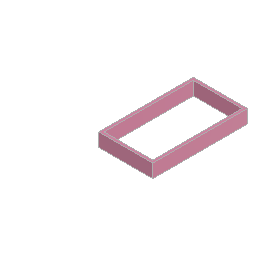
Digital-Storage-Holdster (Autodesk Fusion 360 design; units mm, degrees)
Autodesk Fusion 360 part; units mm, degrees
sketch "Sketch1" plane through (0, 0, 3.175) normal (0, 0, 1) x (-1, 0, 0)
  line L0 (0, 0) -> (0, 297.942)
  line L1 (0, 297.942) -> (-407.924, 297.942)
  line L2 (-407.924, 297.942) -> (-407.924, 0)
  line L3 (-407.924, 0) -> (0, 0)
  line L4 (0, 297.942) -> (-60, 297.942)
  line L5 (-60, 297.942) -> (-60, 192.942)
  line L6 (-60, 192.942) -> (0, 192.942)
  line L7 (0, 192.942) -> (0, 297.942)
  line L8 (-2.95, 294.992) -> (-57.05, 294.992)
  line L9 (-57.05, 294.992) -> (-57.05, 195.892)
  line L10 (-57.05, 195.892) -> (-2.95, 195.892)
  line L11 (-2.95, 195.892) -> (-2.95, 294.992)
  point P0 (0, 297.942)
  dimension "d1" = 60
  dimension "d2" = 105
  constraint horizontal L4
  constraint vertical L5
  constraint horizontal L6
  constraint vertical L7
  constraint coincident P0 L0.end
  measures "d1" distance of P0 L4.end
  measures "d2" distance of P0 L6.end
extrude "Extrude1" add sketch "Sketch1" along normal blind 15 contours L0 L1 L4 L5 L6 L7
equation "d1 = OnlineStorageWidth"
equation "d2 = OnlineStorageLength"
equation "d5 = -HoldersterWallWidth + SmallTolerence"
equation "d9 = HoldersterHeightLow"
equation "SmallTolerence = 0.05 mm"
equation "HoldersterWallWidth = 3 mm"
equation "OnlineStorageLength = 105 mm"
equation "OnlineStorageWidth = 60 mm"
equation "HoldersterHeightLow = 15 mm"
